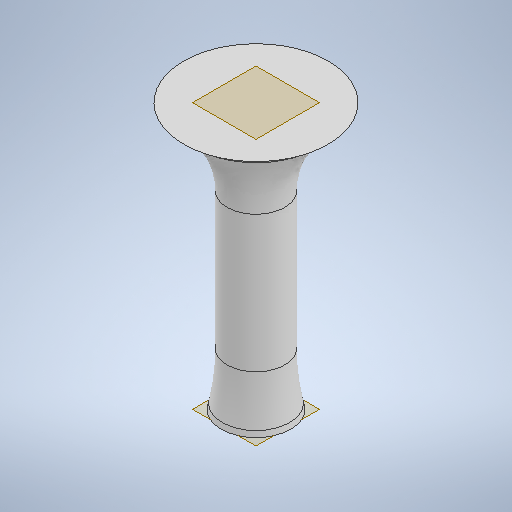
# Autodesk Inventor part: table_column
Saved by Autodesk Inventor 2025.2 (Build 292293000, 293)
## iProperties
Created: 2024-12-28
Part Number: table_column
Material: Generic
Document SubType Name: Modeling
Designer: holz
Density: 1 g/cm^3
Appearance: Default
Author: holz
Autodesk Inventor part; units mm, degrees
ref_plane "YZ Plane" through (0, 0, 0) normal (1, 0, 0) x (0, 1, 0)
ref_plane "XY Plane" through (0, 0, 0) normal (0, 0, 1) x (1, 0, 0)
sketch "Sketch1" plane through (0, 0, 0) normal (0, 1, 0) x (-1, 0, 0)
  circle A0 centre (0, 0) radius 5
  dimension "d0" = 10
  constraints: 1 centre point, 1 coincident
  measures "d0" diameter of A0
extrude "Extrusion1" add sketch "Sketch1" along normal blind 35
ref_plane "Work Plane1" through (0, -5, 0) normal (0, 1, 0) x (-1, 0, 0)
sketch "Sketch4" plane through (0, -5, 0) normal (0, 1, 0) x (-1, 0, 0)
  circle A0 centre (0, 0) radius 6
  dimension "d8" = 12
  constraints: 1 centre point, 1 coincident
  measures "d8" diameter of A0
loft "Loft1" add profiles "Sketch4" section 1 edges at (5, 0, 0)
ref_plane "Work Plane2" through (0, 41, 0) normal (0, 1, 0) x (1, 0, 0)
sketch "Sketch5" plane through (0, 41, 0) normal (0, 1, 0) x (1, 0, 0)
  circle A0 centre (0, 0) radius 12.5
  dimension "d14" = 25
  constraints: 1 centre point, 1 coincident
  measures "d14" diameter of A0
loft "Loft2" add profiles "Sketch5" section 2 edges at (5, 35, 0)
fillet "Face Fillet1" radius 15 2 edges at (0, 35, -5) (0, 35, 5)
fillet "Face Fillet2" radius 42 1 edges at (5, 0, 0)
body "Solid1"
